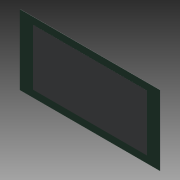
# Autodesk Inventor part: Arena Base
Saved by Autodesk Inventor 2013 (Build 170138000, 138)
## iProperties
Created: 2013-01-07
Part Number: Arena Base
Material: Generic
Document SubType Name: Modeling
Designer: Phillip
Density: 1 g/cm^3
Author: Phillip
Autodesk Inventor part; units mm, degrees
ref_plane "YZ Plane" through (0, 0, 0) normal (1, 0, 0) x (0, 1, 0)
ref_plane "XZ Plane" through (0, 0, 0) normal (0, 1, 0) x (-1, 0, 0)
ref_plane "XY Plane" through (0, 0, 0) normal (0, 0, 1) x (1, 0, 0)
sketch "Sketch1" plane through (0, 0, 0) normal (0, 0, 1) x (1, 0, 0)
  line L0 (0, 0) -> (20320, 0)
  line L1 (20320, 0) -> (20320, 10160)
  line L2 (20320, 10160) -> (0, 10160)
  line L3 (0, 10160) -> (0, 0)
  dimension "d0" = 20320
  dimension "d1" = 10160
  constraints: 8 end point, 2 parallel, 1 horizontal, 1 perpendicular
  measures "d0" distance of L2.end L1.end
  measures "d1" distance of L1.end L0.end
extrude "Extrusion1" add sketch "Sketch1" against normal blind 25.4
sketch "Sketch2" plane through (0, 0, 0) normal (0, 0, 1) x (1, 0, 0)
  line L0 (20320, 10160) -> (0, 10160) projected
  line L1 (0, 10160) -> (0, 0) projected
  line L2 (1911.604, 997.331) -> (18408.396, 997.331)
  line L3 (18408.396, 997.331) -> (18408.396, 9162.669)
  line L4 (18408.396, 9162.669) -> (1911.604, 9162.669)
  line L5 (1911.604, 9162.669) -> (1911.604, 997.331)
  point P0 (1911.604, 5080)
  point P1 (0, 5080)
  point P2 (10160, 9162.669)
  point P3 (10160, 10160)
  dimension "d4" = 16496.792
  dimension "d6" = 8165.338
  constraints: 8 end point, 4 midpoint, 2 parallel, 1 horizontal, 1 horizontal alignment, 1 perpendicular, 1 vertical alignment
  measures "d4" distance of L3.end L4.end
  measures "d6" distance of L4.end L2.start
extrude "Extrusion2" add sketch "Sketch2" along normal blind 2.54
body "Solid1"
